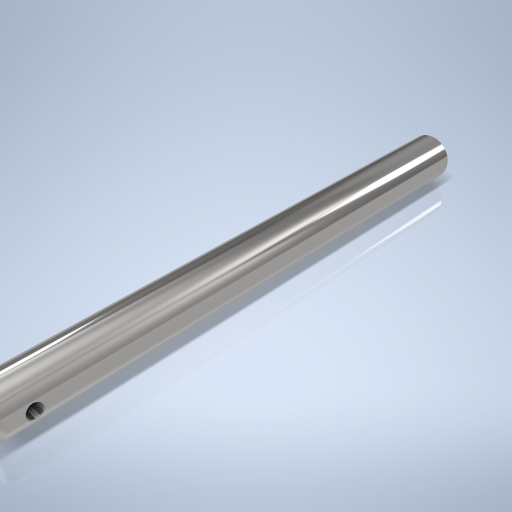
# Autodesk Inventor part: BMS_fiiting_long
Saved by Autodesk Inventor 2024.2 (Build 282272000, 272)
## iProperties
Created: 2024-05-14
Part Number: BMS_fiiting_long
Material: Edelstahl
Document SubType Name: Modeling
Designer: Fabri
Density: 8 g/cm^3
Appearance: Kordiert 45
Author: Fabri
Autodesk Inventor part; units mm, degrees
ref_plane "XZ Plane" through (0, 0, 0) normal (0, 1, 0) x (-1, 0, 0)
ref_plane "XY Plane" through (0, 0, 0) normal (0, 0, 1) x (1, 0, 0)
sketch "Skizze1" plane through (0, 0, 0) normal (0, 1, 0) x (-1, 0, 0)
  circle A0 centre (0, 0) radius 3.25
  dimension "d0" = 6.5
  constraints: 1 centre point, 1 coincident
  measures "d0" diameter of A0
extrude "Extrusion1" add sketch "Skizze1" along normal blind 73
chamfer "Fasen1" distance 0.8 angle 45 2 edges at (3.25, 73, 0) (3.25, 0, 0)
ref_plane "Arbeitsebene1" through (3.25, 0, 0) normal (1, 0, 0) x (0, 1, 0)
sketch "Skizze2" plane through (3.25, 0, 0) normal (1, 0, 0) x (0, 1, 0)
  point P0 (0, 0)
  point P1 (4, 0)
  dimension "d7" = 4
  constraints: 1 horizontal alignment
  measures "d7" distance of point (0, 0) point (4, 0)
hole "Bohrung1" at (3.25, 4, 0) direction (-1, 0, 0) diameter 2 end through all
